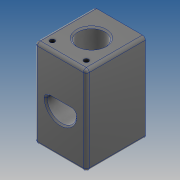
# Autodesk Inventor part: 103.003.01_Gehaeuse_Granulatfuehrung
Saved by Autodesk Inventor 2021 (Build 250183000, 183)
## iProperties
Created: 2020-11-30
Part Number: 103.003.01_Gehaeuse_Granulatfuehrung
Material: Polypropylen
Document SubType Name: Modeling
Designer: Alexander Fritzsche
Density: 0.899 g/cm^3
Appearance: Glatt - Esche
Mass: 60.8448 g
Surface Area: 149.649 cm^2
Volume: 67.6805 cm^3
Author: Alexander Fritzsche
Title: Granulatfuehrung
Autodesk Inventor part; units mm, degrees
ref_plane "YZ Plane" through (0, 0, 0) normal (1, 0, 0) x (0, 1, 0)
ref_plane "XZ Plane" through (0, 0, 0) normal (0, 1, 0) x (-1, 0, 0)
ref_plane "XY Plane" through (0, 0, 0) normal (0, 0, 1) x (1, 0, 0)
sketch "Sketch1" plane through (0, 0, 0) normal (0, 0, 1) x (1, 0, 0)
  line L0 (-17.5, 30) -> (17.5, 30)
  line L1 (17.5, 30) -> (17.5, -30)
  line L2 (17.5, -30) -> (-17.5, -30)
  line L3 (-17.5, -30) -> (-17.5, 30)
  line L4 (0, 9.3667) -> (0, 0)
  line L5 (0, 0) -> (7.7585, 0)
  dimension "d0" = 35
  dimension "d1" = 60
  constraints: 12 end point, 2 parallel, 2 perpendicular, 1 horizontal, 1 vertical, 2 other
  measures "d0" distance of L0.start L0.end
  measures "d1" distance of L0.end L1.end
extrude "Extrusion1" add sketch "Sketch1" along normal blind 40
sketch "Sketch2" plane through (0, 0, 40) normal (0, 0, 1) x (1, 0, 0)
  arc A0 (-10, 0) -> (10, 0) centre (0, 0) ccw
  line L0 (-17.5, -30) -> (17.5, -30) projected
  line L1 (-10, 0) -> (-10, 2.5)
  line L2 (-10, 2.5) -> (10, 2.5)
  line L3 (10, 2.5) -> (10, 0)
  dimension "d8" = 2.5
  dimension "d9" = 20
  dimension "d80" = 10
  constraints: 6 end point, 2 perpendicular, 2 point on circle, 2 tangent, 1 centre point, 1 coincident, 1 vertical
  measures "d8" distance from line of L2 point (0, 0)
  measures "d9" distance of L1.end L2.end
  measures "d80" radius of A0
extrude "Extrusion2" cut sketch "Sketch2" against normal up to surface (40 mm away)
fillet "Fillet1" radius 2.5 2 edges at (-10, 2.5, 20) (10, 2.5, 20)
sketch "Sketch6" plane through (-17.5, -30, 0) normal (0, -1, 0) x (1, 0, 0)
  line L0 (17.5, 0) -> (17.5, 25.5492)
  line L1 (0, 0) -> (0, 40) construction
  line L2 (0, 40) -> (35, 40) projected
  line L3 (35, 0) -> (35, 40) projected
  point P0 (6, 34)
  point P1 (29, 34)
  dimension "d139" = 6
  dimension "d140" = 6
  dimension "d164" = 6
  dimension "d165" = 6
  constraints: 2 end point, 1 horizontal alignment, 1 vertical
  measures "d139" distance from line of L2 point (6, 34)
  measures "d140" distance from line of L1 point (6, 34)
  measures "d164" distance from line of L2 point (29, 34)
  measures "d165" distance from line of L3 point (29, 34)
hole "Hole4" at (-11.5, -30, 34) at (11.5, -30, 34) direction (0, 1, 0) diameter 3.242 depth 12 tip angle 118 thread size "M4x0.7" class "6H" standard "ISO Metric profile"
mirror "Spiegeln3" about plane through (0, 0, 0) normal (0, 1, 0) of "Hole4"
fillet "Rundung2" radius 2 8 edges at (17.5, 30, 20) (0, 30, 40) (17.5, 0, 40) (-17.5, 30, 20) (17.5, -30, 20) (-17.5, -30, 20) (0, -30, 40) (-17.5, 0, 40)
sketch "Skizze23" plane through (-15.5, 30, 0) normal (0, 1, 0) x (1, 0, 0)
  circle A0 centre (15.5, -19) radius 9.1
  line L0 (0, -40) -> (31, -40) projected
  line L1 (-2, 0) -> (-2, -38) projected
  point P0 (15.5, 0)
  dimension "d173" = 18.2
  dimension "d174" = 21
  dimension "d175" = 17.5
  constraints: 1 centre point
  measures "d173" diameter of A0
  measures "d174" distance from line of L0 A0.centre
  measures "d175" distance from line of L1 A0.centre
extrude "Extrusion14" cut sketch "Skizze23" against normal up to surface
chamfer "Fase1" distance 1 angle 45 14 edges at (-9.1, 30, 19) (0, -10, 0) (9.2679, 1.7679, 0) (0, 2.5, 0) (-9.2679, 1.7679, 0) (0, -10, 40) (-9.2679, 1.7679, 40) (0, 2.5, 40) (9.2679, 1.7679, 40) (0, 2.5, 9.9) (0, 2.5, 28.1) (8.7024, 2.1921, 16.3395) (8.7024, 2.1921, 21.6605) (-9.1, 1.9212, 18.9844)
sketch "Skizze25" plane through (0, 0, 0) normal (0, 0, -1) x (-1, 0, 0)
  line L0 (-17.5, -28) -> (-17.5, 28) projected
  line L1 (15.5, -30) -> (-15.5, -30) projected
  line L2 (17.5, 28) -> (17.5, -28) projected
  line L3 (-15.5, 30) -> (15.5, 30) projected
  point P0 (0, 0)
  point P1 (-11.5, -24)
  point P2 (-11.5, 24)
  point P3 (11.5, 24)
  point P4 (11.5, -24)
  dimension "d191" = 6
  dimension "d192" = 6
  dimension "d193" = 6
  dimension "d194" = 6
  constraints: 2 horizontal alignment, 2 vertical alignment
  measures "d191" distance from line of L0 point (-11.5, -24)
  measures "d192" distance from line of L1 point (-11.5, -24)
  measures "d193" distance from line of L2 point (11.5, -24)
  measures "d194" distance from line of L3 point (-11.5, 24)
hole "Bohrung5" at (11.5, -24, 0) at (11.5, 24, 0) at (-11.5, 24, 0) at (-11.5, -24, 0) direction (0, 0, 1) diameter 2.459 depth 8.8 tip angle 118 thread size "M3x0.5" class "6H" standard "ISO Metric profile"
body "Solid1"
